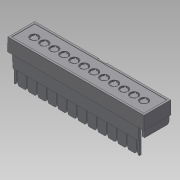
# Autodesk Inventor part: D2MG guard
Saved by Autodesk Inventor 2018.2 (Build 222227000, 227)
## iProperties
Created: 2015-02-09
Part Number: D2MG guard
Material: Типовые
Document SubType Name: Modeling
Designer: Abbath
Density: 1 g/cm^3
Appearance: По умолчанию
Mass: 2.0666 g
Surface Area: 34.2818 cm^2
Volume: 2.0666 cm^3
Author: Abbath
Autodesk Inventor part; units mm, degrees
ref_plane "YZ Plane" through (0, 0, 0) normal (1, 0, 0) x (0, 1, 0)
ref_plane "XZ Plane" through (0, 0, 0) normal (0, 1, 0) x (-1, 0, 0)
sketch "Эскиз1" plane through (0, 0, 0) normal (0, 0, 1) x (1, 0, 0)
  line L0 (-34.8, 6.95) -> (34.8, 6.95)
  line L1 (34.8, 6.95) -> (34.8, -6.95)
  line L2 (34.8, -6.95) -> (-34.8, -6.95)
  line L3 (-34.8, -6.95) -> (-34.8, 6.95)
  point P0 (0, 0)
  point P1 (34.8, 0)
  point P2 (0, 6.95)
  dimension "d0" = 13.9
  dimension "d1" = 69.6
  constraints: 8 end point, 2 midpoint, 2 parallel, 1 horizontal, 1 horizontal alignment, 1 perpendicular, 1 vertical alignment
  measures "d0" distance between parallel lines of L2 L0
  measures "d1" distance between parallel lines of L1 L3
ref_plane "РабПлоскость1" through (0, 0, 6.5) normal (0, 0, 1) x (1, 0, 0)
sketch "Эскиз2" plane through (0, 0, 6.5) normal (0, 0, 1) x (1, 0, 0)
  line L0 (-34.685, 6.85) -> (34.685, 6.85)
  line L1 (34.685, 6.85) -> (34.685, -6.95)
  line L2 (34.685, -6.95) -> (-34.685, -6.95)
  line L3 (-34.685, -6.95) -> (-34.685, 6.85)
  line L4 (34.8, -6.95) -> (-34.8, -6.95) projected
  point P0 (0, 0)
  point P1 (0, 6.85)
  point P2 (0, -6.95)
  dimension "d3" = 13.8
  dimension "d4" = 69.37
  constraints: 8 end point, 2 midpoint, 2 parallel, 1 collinear, 1 horizontal, 1 perpendicular, 1 vertical alignment
  measures "d3" distance between parallel lines of L2 L0
  measures "d4" distance between parallel lines of L1 L3
loft "Лофт1" add profiles "Эскиз1", "Эскиз2"
sketch "Эскиз3" plane through (-34.8, -6.95, 0) normal (0, -1, 0) x (1, 0, 0)
  line L0 (32.55, 7.5) -> (37.05, 7.5)
  line L1 (37.05, 7.5) -> (37.05, 1)
  line L2 (37.05, 1) -> (32.55, 1)
  line L3 (32.55, 1) -> (32.55, 7.5)
  line L4 (69.6, 0) -> (0, 0) projected
  line L5 (69.485, 6.5) -> (0.115, 6.5) construction
  point P0 (34.8, 0)
  point P1 (34.8, 1)
  point P2 (34.8, 0)
  dimension "d9" = 1
  dimension "d10" = 5.5
  dimension "d11" = 4.5
  constraints: 8 end point, 2 midpoint, 2 parallel, 1 horizontal, 1 perpendicular, 1 vertical alignment
  measures "d9" distance between parallel lines of L5 L0
  measures "d10" distance between parallel lines of L2 L5
  measures "d11" distance between parallel lines of L1 L3
extrude "Выдавливание1" cut sketch "Эскиз3" against normal blind 0.5
sketch "Эскиз4" plane through (-34.685, 6.85, 6.5) normal (0, 0, 1) x (1, 0, 0)
  line L0 (32.435, -13.8) -> (32.435, -13.3) construction
  line L1 (32.435, -13.3) -> (36.935, -13.3) construction
  line L2 (36.935, -13.3) -> (36.935, -13.8) construction
  line L3 (69.37, -13.8) -> (36.935, -13.8) construction
  line L4 (69.37, 0) -> (69.37, -13.8) construction
  line L5 (0, 0) -> (69.37, 0) construction
  line L6 (0, -13.8) -> (0, 0) construction
  line L7 (32.435, -13.8) -> (0, -13.8) construction
  line L8 (32.435, -13.8) -> (32.435, -13.3) construction
  line L9 (32.435, -13.3) -> (36.935, -13.3) construction
  line L10 (36.935, -13.3) -> (36.935, -13.8) construction
  line L11 (69.37, -13.8) -> (36.935, -13.8) construction
  line L12 (69.37, 0) -> (69.37, -13.8) construction
  line L13 (0, 0) -> (69.37, 0) construction
  line L14 (0, -13.8) -> (0, 0) construction
  line L15 (32.435, -13.8) -> (0, -13.8) construction
  line L16 (1, -1) -> (68.37, -1)
  line L17 (68.37, -1) -> (68.37, -12.8)
  line L18 (68.37, -12.8) -> (1, -12.8)
  line L19 (1, -12.8) -> (1, -1)
  dimension "d103" = 1
  dimension "d104" = 1
  dimension "d105" = 1
  dimension "d106" = 1
  constraints: 8 end point, 2 parallel, 1 horizontal, 1 perpendicular
  measures "d103" distance between parallel lines of L6 L19
  measures "d104" distance between parallel lines of L4 L17
  measures "d105" distance between parallel lines of L5 L16
  measures "d106" distance between parallel lines of L3 L18
extrude "Выдавливание2" cut sketch "Эскиз4" against normal blind 0.2
sketch "Эскиз5" plane through (-34.685, 6.85, 6.3) normal (0, 0, 1) x (1, 0, 0)
  line L0 (-0.115, 0.1) -> (69.485, 0.1) construction
  line L1 (34.685, 0.1) -> (34.685, -13.8) construction
  line L2 (69.485, -13.8) -> (-0.115, -13.8) construction
  line L3 (34.685, -6.85) -> (81.7504, -6.85) construction
  circle A0 centre (37.225, -6.85) radius 2.1
  circle A1 centre (42.305, -6.85) radius 2.1
  circle A2 centre (47.385, -6.85) radius 2.1
  circle A3 centre (52.465, -6.85) radius 2.1
  circle A4 centre (57.545, -6.85) radius 2.1
  circle A5 centre (62.625, -6.85) radius 2.1
  circle A6 centre (32.145, -6.85) radius 2.1
  circle A7 centre (37.225, -6.85) radius 2.1
  circle A8 centre (42.305, -6.85) radius 2.1
  circle A9 centre (47.385, -6.85) radius 2.1
  circle A10 centre (52.465, -6.85) radius 2.1
  circle A11 centre (57.545, -6.85) radius 2.1
  circle A12 centre (27.065, -6.85) radius 2.1
  circle A13 centre (32.145, -6.85) radius 2.1
  circle A14 centre (37.225, -6.85) radius 2.1
  circle A15 centre (42.305, -6.85) radius 2.1
  circle A16 centre (47.385, -6.85) radius 2.1
  circle A17 centre (52.465, -6.85) radius 2.1
  circle A18 centre (21.985, -6.85) radius 2.1
  circle A19 centre (27.065, -6.85) radius 2.1
  circle A20 centre (32.145, -6.85) radius 2.1
  circle A21 centre (37.225, -6.85) radius 2.1
  circle A22 centre (42.305, -6.85) radius 2.1
  circle A23 centre (47.385, -6.85) radius 2.1
  circle A24 centre (16.905, -6.85) radius 2.1
  circle A25 centre (21.985, -6.85) radius 2.1
  circle A26 centre (27.065, -6.85) radius 2.1
  circle A27 centre (32.145, -6.85) radius 2.1
  circle A28 centre (37.225, -6.85) radius 2.1
  circle A29 centre (42.305, -6.85) radius 2.1
  circle A30 centre (11.825, -6.85) radius 2.1
  circle A31 centre (16.905, -6.85) radius 2.1
  circle A32 centre (21.985, -6.85) radius 2.1
  circle A33 centre (27.065, -6.85) radius 2.1
  circle A34 centre (32.145, -6.85) radius 2.1
  circle A35 centre (37.225, -6.85) radius 2.1
  circle A36 centre (6.745, -6.85) radius 2.1
  circle A37 centre (11.825, -6.85) radius 2.1
  circle A38 centre (16.905, -6.85) radius 2.1
  circle A39 centre (21.985, -6.85) radius 2.1
  circle A40 centre (27.065, -6.85) radius 2.1
  circle A41 centre (32.145, -6.85) radius 2.1
  line L4 (32.145, -6.85) -> (37.225, -6.85) construction
  dimension "d107" = 4.2
  dimension "d110" = 5.08
  dimension "d113" = 5.08
  constraints: 42 centre point, 6 end point, 5 midpoint, 3 horizontal, 1 collinear, 1 point on line, 82 other
  measures "d107" diameter of A0
  measures "d110" distance of A0.centre A1.centre
  measures "d113" distance of A0.centre A6.centre
extrude "Выдавливание3" cut sketch "Эскиз5" against normal blind 0.3
sketch "Эскиз6" plane through (-12.7, 0, 6) normal (0, 0, 1) x (1, 0, 0)
  circle A0 centre (-15.24, 0) radius 2.1 construction
  circle A1 centre (-15.24, 0) radius 2.1 projected
  line L0 (-17.3106, 0.35) -> (-16.6986, 0.35)
  line L1 (-17.3106, -0.35) -> (-16.6986, -0.35)
  line L2 (-15.24, 0) -> (-17.34, 0) construction
  line L3 (-17.0605, 0.35) -> (-17.0605, -0.35) construction
  line L4 (-14.5078, -1.9682) -> (-14.8138, -1.4382)
  line L5 (-13.9016, -1.6182) -> (-14.2076, -1.0882)
  line L6 (-13.9016, 1.6182) -> (-14.2076, 1.0882)
  line L7 (-14.5078, 1.9682) -> (-14.8138, 1.4382)
  arc A2 (-14.8138, 1.4382) -> (-16.6986, 0.35) centre (-15.24, 0) ccw
  arc A3 (-14.5078, 1.9682) -> (-17.3106, 0.35) centre (-15.24, 0) ccw
  arc A4 (-17.3106, -0.35) -> (-14.5078, -1.9682) centre (-15.24, 0) ccw
  arc A5 (-13.9016, -1.6182) -> (-13.9016, 1.6182) centre (-15.24, 0) ccw
  arc A6 (-16.6986, -0.35) -> (-14.8138, -1.4382) centre (-15.24, 0) ccw
  arc A7 (-14.2076, -1.0882) -> (-14.2076, 1.0882) centre (-15.24, 0) ccw
  line L8 (-9.4278, 1.9682) -> (-9.7338, 1.4382)
  line L9 (-9.4278, -1.9682) -> (-9.7338, -1.4382)
  arc A8 (-9.7338, 1.4382) -> (-11.6186, 0.35) centre (-10.16, 0) ccw
  arc A9 (-9.4278, 1.9682) -> (-12.2306, 0.35) centre (-10.16, 0) ccw
  arc A10 (-11.6186, -0.35) -> (-9.7338, -1.4382) centre (-10.16, 0) ccw
  arc A11 (-12.2306, -0.35) -> (-9.4278, -1.9682) centre (-10.16, 0) ccw
  line L10 (-10.16, 0) -> (-12.26, 0) construction
  line L11 (-11.9805, 0.35) -> (-11.9805, -0.35) construction
  line L12 (-12.2306, -0.35) -> (-11.6186, -0.35)
  line L13 (-12.2306, 0.35) -> (-11.6186, 0.35)
  line L14 (-8.8216, -1.6182) -> (-9.1276, -1.0882)
  arc A12 (-9.1276, -1.0882) -> (-9.1276, 1.0882) centre (-10.16, 0) ccw
  arc A13 (-8.8216, -1.6182) -> (-8.8216, 1.6182) centre (-10.16, 0) ccw
  line L15 (-8.8216, 1.6182) -> (-9.1276, 1.0882)
  line L16 (-4.3478, 1.9682) -> (-4.6538, 1.4382)
  line L17 (-4.3478, -1.9682) -> (-4.6538, -1.4382)
  arc A14 (-4.6538, 1.4382) -> (-6.5386, 0.35) centre (-5.08, 0) ccw
  arc A15 (-4.3478, 1.9682) -> (-7.1506, 0.35) centre (-5.08, 0) ccw
  arc A16 (-6.5386, -0.35) -> (-4.6538, -1.4382) centre (-5.08, 0) ccw
  arc A17 (-7.1506, -0.35) -> (-4.3478, -1.9682) centre (-5.08, 0) ccw
  line L18 (-5.08, 0) -> (-7.18, 0) construction
  line L19 (-6.9005, 0.35) -> (-6.9005, -0.35) construction
  line L20 (-7.1506, -0.35) -> (-6.5386, -0.35)
  line L21 (-7.1506, 0.35) -> (-6.5386, 0.35)
  line L22 (-3.7416, -1.6182) -> (-4.0476, -1.0882)
  arc A18 (-4.0476, -1.0882) -> (-4.0476, 1.0882) centre (-5.08, 0) ccw
  arc A19 (-3.7416, -1.6182) -> (-3.7416, 1.6182) centre (-5.08, 0) ccw
  line L23 (-3.7416, 1.6182) -> (-4.0476, 1.0882)
  line L24 (0.7322, 1.9682) -> (0.4262, 1.4382)
  line L25 (0.7322, -1.9682) -> (0.4262, -1.4382)
  arc A20 (0.4262, 1.4382) -> (-1.4586, 0.35) centre (0, 0) ccw
  arc A21 (0.7322, 1.9682) -> (-2.0706, 0.35) centre (0, 0) ccw
  arc A22 (-1.4586, -0.35) -> (0.4262, -1.4382) centre (0, 0) ccw
  arc A23 (-2.0706, -0.35) -> (0.7322, -1.9682) centre (0, 0) ccw
  line L26 (0, 0) -> (-2.1, 0) construction
  line L27 (-1.8205, 0.35) -> (-1.8205, -0.35) construction
  line L28 (-2.0706, -0.35) -> (-1.4586, -0.35)
  line L29 (-2.0706, 0.35) -> (-1.4586, 0.35)
  line L30 (1.3384, -1.6182) -> (1.0324, -1.0882)
  arc A24 (1.0324, -1.0882) -> (1.0324, 1.0882) centre (0, 0) ccw
  arc A25 (1.3384, -1.6182) -> (1.3384, 1.6182) centre (0, 0) ccw
  line L31 (1.3384, 1.6182) -> (1.0324, 1.0882)
  line L32 (5.8122, 1.9682) -> (5.5062, 1.4382)
  line L33 (5.8122, -1.9682) -> (5.5062, -1.4382)
  arc A26 (5.5062, 1.4382) -> (3.6214, 0.35) centre (5.08, 0) ccw
  arc A27 (5.8122, 1.9682) -> (3.0094, 0.35) centre (5.08, 0) ccw
  arc A28 (3.6214, -0.35) -> (5.5062, -1.4382) centre (5.08, 0) ccw
  arc A29 (3.0094, -0.35) -> (5.8122, -1.9682) centre (5.08, 0) ccw
  line L34 (5.08, 0) -> (2.98, 0) construction
  line L35 (3.2595, 0.35) -> (3.2595, -0.35) construction
  line L36 (3.0094, -0.35) -> (3.6214, -0.35)
  line L37 (3.0094, 0.35) -> (3.6214, 0.35)
  line L38 (6.4184, -1.6182) -> (6.1124, -1.0882)
  arc A30 (6.1124, -1.0882) -> (6.1124, 1.0882) centre (5.08, 0) ccw
  arc A31 (6.4184, -1.6182) -> (6.4184, 1.6182) centre (5.08, 0) ccw
  line L39 (6.4184, 1.6182) -> (6.1124, 1.0882)
  line L40 (10.8922, 1.9682) -> (10.5862, 1.4382)
  line L41 (10.8922, -1.9682) -> (10.5862, -1.4382)
  arc A32 (10.5862, 1.4382) -> (8.7014, 0.35) centre (10.16, 0) ccw
  arc A33 (10.8922, 1.9682) -> (8.0894, 0.35) centre (10.16, 0) ccw
  arc A34 (8.7014, -0.35) -> (10.5862, -1.4382) centre (10.16, 0) ccw
  arc A35 (8.0894, -0.35) -> (10.8922, -1.9682) centre (10.16, 0) ccw
  line L42 (10.16, 0) -> (8.06, 0) construction
  line L43 (8.3395, 0.35) -> (8.3395, -0.35) construction
  line L44 (8.0894, -0.35) -> (8.7014, -0.35)
  line L45 (8.0894, 0.35) -> (8.7014, 0.35)
  line L46 (11.4984, -1.6182) -> (11.1924, -1.0882)
  arc A36 (11.1924, -1.0882) -> (11.1924, 1.0882) centre (10.16, 0) ccw
  arc A37 (11.4984, -1.6182) -> (11.4984, 1.6182) centre (10.16, 0) ccw
  line L47 (11.4984, 1.6182) -> (11.1924, 1.0882)
  line L48 (15.9722, 1.9682) -> (15.6662, 1.4382)
  line L49 (15.9722, -1.9682) -> (15.6662, -1.4382)
  arc A38 (15.6662, 1.4382) -> (13.7814, 0.35) centre (15.24, 0) ccw
  arc A39 (15.9722, 1.9682) -> (13.1694, 0.35) centre (15.24, 0) ccw
  arc A40 (13.7814, -0.35) -> (15.6662, -1.4382) centre (15.24, 0) ccw
  arc A41 (13.1694, -0.35) -> (15.9722, -1.9682) centre (15.24, 0) ccw
  line L50 (15.24, 0) -> (13.14, 0) construction
  line L51 (13.4195, 0.35) -> (13.4195, -0.35) construction
  line L52 (13.1694, -0.35) -> (13.7814, -0.35)
  line L53 (13.1694, 0.35) -> (13.7814, 0.35)
  line L54 (16.5784, -1.6182) -> (16.2724, -1.0882)
  arc A42 (16.2724, -1.0882) -> (16.2724, 1.0882) centre (15.24, 0) ccw
  arc A43 (16.5784, -1.6182) -> (16.5784, 1.6182) centre (15.24, 0) ccw
  line L55 (16.5784, 1.6182) -> (16.2724, 1.0882)
  line L56 (21.0522, 1.9682) -> (20.7462, 1.4382)
  line L57 (21.0522, -1.9682) -> (20.7462, -1.4382)
  arc A44 (20.7462, 1.4382) -> (18.8614, 0.35) centre (20.32, 0) ccw
  arc A45 (21.0522, 1.9682) -> (18.2494, 0.35) centre (20.32, 0) ccw
  arc A46 (18.8614, -0.35) -> (20.7462, -1.4382) centre (20.32, 0) ccw
  arc A47 (18.2494, -0.35) -> (21.0522, -1.9682) centre (20.32, 0) ccw
  line L58 (20.32, 0) -> (18.22, 0) construction
  line L59 (18.4995, 0.35) -> (18.4995, -0.35) construction
  line L60 (18.2494, -0.35) -> (18.8614, -0.35)
  line L61 (18.2494, 0.35) -> (18.8614, 0.35)
  line L62 (21.6584, -1.6182) -> (21.3524, -1.0882)
  arc A48 (21.3524, -1.0882) -> (21.3524, 1.0882) centre (20.32, 0) ccw
  arc A49 (21.6584, -1.6182) -> (21.6584, 1.6182) centre (20.32, 0) ccw
  line L63 (21.6584, 1.6182) -> (21.3524, 1.0882)
  line L64 (26.1322, 1.9682) -> (25.8262, 1.4382)
  line L65 (26.1322, -1.9682) -> (25.8262, -1.4382)
  arc A50 (25.8262, 1.4382) -> (23.9414, 0.35) centre (25.4, 0) ccw
  arc A51 (26.1322, 1.9682) -> (23.3294, 0.35) centre (25.4, 0) ccw
  arc A52 (23.9414, -0.35) -> (25.8262, -1.4382) centre (25.4, 0) ccw
  arc A53 (23.3294, -0.35) -> (26.1322, -1.9682) centre (25.4, 0) ccw
  line L66 (25.4, 0) -> (23.3, 0) construction
  line L67 (23.5795, 0.35) -> (23.5795, -0.35) construction
  line L68 (23.3294, -0.35) -> (23.9414, -0.35)
  line L69 (23.3294, 0.35) -> (23.9414, 0.35)
  line L70 (26.7384, -1.6182) -> (26.4324, -1.0882)
  arc A54 (26.4324, -1.0882) -> (26.4324, 1.0882) centre (25.4, 0) ccw
  arc A55 (26.7384, -1.6182) -> (26.7384, 1.6182) centre (25.4, 0) ccw
  line L71 (26.7384, 1.6182) -> (26.4324, 1.0882)
  line L72 (31.2122, 1.9682) -> (30.9062, 1.4382)
  line L73 (31.2122, -1.9682) -> (30.9062, -1.4382)
  arc A56 (30.9062, 1.4382) -> (29.0214, 0.35) centre (30.48, 0) ccw
  arc A57 (31.2122, 1.9682) -> (28.4094, 0.35) centre (30.48, 0) ccw
  arc A58 (29.0214, -0.35) -> (30.9062, -1.4382) centre (30.48, 0) ccw
  arc A59 (28.4094, -0.35) -> (31.2122, -1.9682) centre (30.48, 0) ccw
  line L74 (30.48, 0) -> (28.38, 0) construction
  line L75 (28.6595, 0.35) -> (28.6595, -0.35) construction
  line L76 (28.4094, -0.35) -> (29.0214, -0.35)
  line L77 (28.4094, 0.35) -> (29.0214, 0.35)
  line L78 (31.8184, -1.6182) -> (31.5124, -1.0882)
  arc A60 (31.5124, -1.0882) -> (31.5124, 1.0882) centre (30.48, 0) ccw
  arc A61 (31.8184, -1.6182) -> (31.8184, 1.6182) centre (30.48, 0) ccw
  line L79 (31.8184, 1.6182) -> (31.5124, 1.0882)
  line L80 (36.2922, 1.9682) -> (35.9862, 1.4382)
  line L81 (36.2922, -1.9682) -> (35.9862, -1.4382)
  arc A62 (35.9862, 1.4382) -> (34.1014, 0.35) centre (35.56, 0) ccw
  arc A63 (36.2922, 1.9682) -> (33.4894, 0.35) centre (35.56, 0) ccw
  arc A64 (34.1014, -0.35) -> (35.9862, -1.4382) centre (35.56, 0) ccw
  arc A65 (33.4894, -0.35) -> (36.2922, -1.9682) centre (35.56, 0) ccw
  line L82 (35.56, 0) -> (33.46, 0) construction
  line L83 (33.7395, 0.35) -> (33.7395, -0.35) construction
  line L84 (33.4894, -0.35) -> (34.1014, -0.35)
  line L85 (33.4894, 0.35) -> (34.1014, 0.35)
  line L86 (36.8984, -1.6182) -> (36.5924, -1.0882)
  arc A66 (36.5924, -1.0882) -> (36.5924, 1.0882) centre (35.56, 0) ccw
  arc A67 (36.8984, -1.6182) -> (36.8984, 1.6182) centre (35.56, 0) ccw
  line L87 (36.8984, 1.6182) -> (36.5924, 1.0882)
  line L88 (41.3722, 1.9682) -> (41.0662, 1.4382)
  line L89 (41.3722, -1.9682) -> (41.0662, -1.4382)
  arc A68 (41.0662, 1.4382) -> (39.1814, 0.35) centre (40.64, 0) ccw
  arc A69 (41.3722, 1.9682) -> (38.5694, 0.35) centre (40.64, 0) ccw
  arc A70 (39.1814, -0.35) -> (41.0662, -1.4382) centre (40.64, 0) ccw
  arc A71 (38.5694, -0.35) -> (41.3722, -1.9682) centre (40.64, 0) ccw
  line L90 (40.64, 0) -> (38.54, 0) construction
  line L91 (38.8195, 0.35) -> (38.8195, -0.35) construction
  line L92 (38.5694, -0.35) -> (39.1814, -0.35)
  line L93 (38.5694, 0.35) -> (39.1814, 0.35)
  line L94 (41.9784, -1.6182) -> (41.6724, -1.0882)
  arc A72 (41.6724, -1.0882) -> (41.6724, 1.0882) centre (40.64, 0) ccw
  arc A73 (41.9784, -1.6182) -> (41.9784, 1.6182) centre (40.64, 0) ccw
  line L95 (41.9784, 1.6182) -> (41.6724, 1.0882)
  point P0 (-17.0605, 0)
  point P1 (-14.6329, -1.7516)
  point P2 (-14.0266, -1.4016)
  point P3 (-14.0266, 1.4016)
  point P4 (-14.6329, 1.7516)
  point P5 (-9.5529, -1.7516)
  point P6 (-9.5529, 1.7516)
  point P7 (-11.9805, 0)
  point P8 (-8.9466, 1.4016)
  point P9 (-8.9466, -1.4016)
  point P10 (-4.4729, -1.7516)
  point P11 (-4.4729, 1.7516)
  point P12 (-6.9005, 0)
  point P13 (-3.8666, 1.4016)
  point P14 (-3.8666, -1.4016)
  point P15 (0.6071, -1.7516)
  point P16 (0.6071, 1.7516)
  point P17 (-1.8205, 0)
  point P18 (1.2134, 1.4016)
  point P19 (1.2134, -1.4016)
  point P20 (5.6871, -1.7516)
  point P21 (5.6871, 1.7516)
  point P22 (3.2595, 0)
  point P23 (6.2934, 1.4016)
  point P24 (6.2934, -1.4016)
  point P25 (10.7671, -1.7516)
  point P26 (10.7671, 1.7516)
  point P27 (8.3395, 0)
  point P28 (11.3734, 1.4016)
  point P29 (11.3734, -1.4016)
  point P30 (15.8471, -1.7516)
  point P31 (15.8471, 1.7516)
  point P32 (13.4195, 0)
  point P33 (16.4534, 1.4016)
  point P34 (16.4534, -1.4016)
  point P35 (20.9271, -1.7516)
  point P36 (20.9271, 1.7516)
  point P37 (18.4995, 0)
  point P38 (21.5334, 1.4016)
  point P39 (21.5334, -1.4016)
  point P40 (26.0071, -1.7516)
  point P41 (26.0071, 1.7516)
  point P42 (23.5795, 0)
  point P43 (26.6134, 1.4016)
  point P44 (26.6134, -1.4016)
  point P45 (31.0871, -1.7516)
  point P46 (31.0871, 1.7516)
  point P47 (28.6595, 0)
  point P48 (31.6934, 1.4016)
  point P49 (31.6934, -1.4016)
  point P50 (36.1671, -1.7516)
  point P51 (36.1671, 1.7516)
  point P52 (33.7395, 0)
  point P53 (36.7734, 1.4016)
  point P54 (36.7734, -1.4016)
  point P55 (41.2471, -1.7516)
  point P56 (41.2471, 1.7516)
  point P57 (38.8195, 0)
  point P58 (41.8534, 1.4016)
  point P59 (41.8534, -1.4016)
  dimension "d117" = 0.7
  dimension "d120" = 360
  dimension "d131" = 5.08
  constraints: 192 end point, 147 point on circle, 84 point on line, 72 centre point, 13 coincident, 3 horizontal, 1 collinear, 1 midpoint, 1 parallel, 1 perpendicular, 431 other
  measures "d117" distance between parallel lines of L1 L0
  measures "d131" distance of A3.centre A9.centre
extrude "Выдавливание4" cut sketch "Эскиз6" against normal through all contours A1 L5 A7 L6 | L7 A2 L0 A1 | A1 L1 A6 L4 | L8 A8 L13 A9 | A11 L12 A10 L9 | L14 A12 L15 A13 | L16 A14 L21 A15 | A17 L20 A16 L17 | L22 A18 L23 A19 | L24 A20 L29 A21 | A23 L28 A22 L25 | L30 A24 L31 A25 | L32 A26 L37 A27 | A29 L36 A28 L33 | L38 A30 L39 A31 | L40 A32 L45 A33 | A35 L44 A34 L41 | L46 A36 L47 A37 | L48 A38 L53 A39 | A41 L52 A40 L49 | L54 A42 L55 A43 | L56 A44 L61 A45 | A47 L60 A46 L57 | L62 A48 L63 A49 | L64 A50 L69 A51 | A53 L68 A52 L65 | L70 A54 L71 A55 | L72 A56 L77 A57 | A59 L76 A58 L73 | L78 A60 L79 A61 | L80 A62 L85 A63 | A65 L84 A64 L81 | L86 A66 L87 A67 | L88 A68 L93 A69 | A71 L92 A70 L89 | L94 A72 L95 A73
sketch "Эскиз7" plane through (34.8, 6.95, 0) normal (0, 0, -1) x (-1, 0, 0)
  line L0 (2.9, 0) -> (66.7, 0)
  line L1 (66.7, 0) -> (66.7, -1.5)
  line L2 (66.7, -1.5) -> (2.9, -1.5)
  line L3 (2.9, -1.5) -> (2.9, 0)
  line L4 (69.6, 0) -> (0, 0) construction
  point P0 (34.8, -6.95)
  point P1 (34.8, -1.5)
  dimension "d39" = 1.5
  dimension "d40" = 63.8
  constraints: 8 end point, 2 parallel, 1 collinear, 1 horizontal, 1 midpoint, 1 perpendicular, 1 vertical alignment
  measures "d39" distance between parallel lines of L2 L4
  measures "d40" distance between parallel lines of L1 L3
extrude "Выдавливание5" add sketch "Эскиз7" along normal blind 12.9
sketch "Эскиз8" plane through (0, 0, 0) normal (1, 0, 0) x (0, 1, 0)
  line L0 (6.33, -12.9) -> (6.42, -5.85)
  line L1 (6.42, -5.85) -> (6.95, -5.85)
  line L2 (5.45, 0) -> (5.45, -12.9) projected
  line L3 (6.95, -5.85) -> (6.95, -12.9)
  line L4 (6.95, -12.9) -> (6.33, -12.9)
  line L5 (6.95, -12.9) -> (5.45, -12.9) construction
  line L6 (6.95, 0) -> (6.95, -12.9) construction
  point P0 (0, 0)
  dimension "d43" = 0.53
  dimension "d44" = 0.88
  dimension "d45" = 7.05
  constraints: 8 end point, 3 perpendicular, 2 collinear
  measures "d43" distance from line of L0.end L3
  measures "d44" distance from line of L0.start L2
  measures "d45" distance from line of L1 L0.start
extrude "Выдавливание6" cut sketch "Эскиз8" along normal through all both and the other way through all
sketch "Эскиз10" plane through (34.8, -6.95, 0) normal (0, 0, -1) x (-1, 0, 0)
  line L0 (67.3, 12.4) -> (2.3, 12.4)
  line L1 (2.3, 12.4) -> (2.3, 1.5)
  line L2 (2.3, 1.5) -> (67.3, 1.5)
  line L3 (67.3, 1.5) -> (67.3, 12.4)
  line L4 (69.6, 0) -> (69.6, 13.9) projected
  line L5 (0, 0) -> (69.6, 0) projected
  line L6 (0, 13.9) -> (0, 0) projected
  line L7 (2.9, 12.4) -> (66.7, 12.4) projected
  point P0 (34.8, 6.95)
  point P1 (45.71, 12.4)
  point P2 (34.8, 1.5)
  dimension "d63" = 1.5
  dimension "d70" = 65
  constraints: 8 end point, 2 parallel, 1 collinear, 1 horizontal, 1 midpoint, 1 perpendicular, 1 vertical alignment
  measures "d63" distance between parallel lines of L5 L2
  measures "d70" distance between parallel lines of L1 L3
extrude "Выдавливание8" cut sketch "Эскиз10" against normal blind 5
sketch "Эскиз17" plane through (-31.9, 6.42, -5.85) normal (0, 0.9999185, -0.0127649) x (1, 0, 0)
  line L0 (0.52, 7.0618) -> (1.17, 5.5381)
  line L1 (1.17, 5.5381) -> (1.17, -0.0455)
  line L2 (1.17, -0.0455) -> (1.67, -0.0455)
  line L3 (1.67, -0.0455) -> (1.67, 5.5381)
  line L4 (1.67, 5.5381) -> (2.32, 7.0618)
  line L5 (0.52, 7.0618) -> (2.32, 7.0618)
  line L6 (1.42, 0) -> (1.42, 8.247) construction
  line L7 (1.17, 0.6294) -> (1.67, 0.6294) construction
  line L8 (0, -5.8371) -> (0, 7.0618) construction
  line L9 (0, 4.1598) -> (63.8, 4.1598) construction
  line L10 (63.8, -5.8371) -> (63.8, 7.0618) construction
  line L11 (31.65, 5.5381) -> (32.15, 5.5381) construction
  line L12 (0.52, 7.0618) -> (2.32, 7.0618) construction
  line L13 (5.6, 7.0618) -> (7.4, 7.0618) construction
  line L14 (10.68, 7.0618) -> (12.48, 7.0618) construction
  line L15 (0.52, 7.0618) -> (2.32, 7.0618) construction
  line L16 (1.17, -0.0455) -> (1.67, -0.0455) construction
  line L17 (63.8, 0) -> (0, 0) projected
  line L18 (1.17, 0) -> (1.67, 0)
  line L19 (6.75, 5.5381) -> (7.4, 7.0618)
  line L20 (5.6, 7.0618) -> (6.25, 5.5381)
  line L21 (5.6, 7.0618) -> (7.4, 7.0618)
  line L22 (5.6, 7.0618) -> (7.4, 7.0618) construction
  line L23 (6.25, 0.6294) -> (6.75, 0.6294) construction
  line L24 (6.75, -0.0455) -> (6.75, 5.5381)
  line L25 (6.25, 5.5381) -> (6.25, -0.0455)
  line L26 (6.25, 0) -> (6.75, 0)
  line L27 (6.25, -0.0455) -> (6.75, -0.0455)
  line L28 (6.25, -0.0455) -> (6.75, -0.0455) construction
  line L29 (36.73, 5.5381) -> (37.23, 5.5381) construction
  line L30 (11.83, 5.5381) -> (12.48, 7.0618)
  line L31 (10.68, 7.0618) -> (11.33, 5.5381)
  line L32 (10.68, 7.0618) -> (12.48, 7.0618)
  line L33 (10.68, 7.0618) -> (12.48, 7.0618) construction
  line L34 (11.33, 0.6294) -> (11.83, 0.6294) construction
  line L35 (11.83, -0.0455) -> (11.83, 5.5381)
  line L36 (11.33, 5.5381) -> (11.33, -0.0455)
  line L37 (11.33, 0) -> (11.83, 0)
  line L38 (11.33, -0.0455) -> (11.83, -0.0455)
  line L39 (11.33, -0.0455) -> (11.83, -0.0455) construction
  line L40 (41.81, 5.5381) -> (42.31, 5.5381) construction
  line L41 (16.91, 5.5381) -> (17.56, 7.0618)
  line L42 (15.76, 7.0618) -> (16.41, 5.5381)
  line L43 (15.76, 7.0618) -> (17.56, 7.0618)
  line L44 (15.76, 7.0618) -> (17.56, 7.0618) construction
  line L45 (16.41, 0.6294) -> (16.91, 0.6294) construction
  line L46 (16.91, -0.0455) -> (16.91, 5.5381)
  line L47 (16.41, 5.5381) -> (16.41, -0.0455)
  line L48 (16.41, 0) -> (16.91, 0)
  line L49 (16.41, -0.0455) -> (16.91, -0.0455)
  line L50 (16.41, -0.0455) -> (16.91, -0.0455) construction
  line L51 (46.89, 5.5381) -> (47.39, 5.5381) construction
  line L52 (21.99, 5.5381) -> (22.64, 7.0618)
  line L53 (20.84, 7.0618) -> (21.49, 5.5381)
  line L54 (20.84, 7.0618) -> (22.64, 7.0618)
  line L55 (20.84, 7.0618) -> (22.64, 7.0618) construction
  line L56 (21.49, 0.6294) -> (21.99, 0.6294) construction
  line L57 (21.99, -0.0455) -> (21.99, 5.5381)
  line L58 (21.49, 5.5381) -> (21.49, -0.0455)
  line L59 (21.49, 0) -> (21.99, 0)
  line L60 (21.49, -0.0455) -> (21.99, -0.0455)
  line L61 (21.49, -0.0455) -> (21.99, -0.0455) construction
  line L62 (51.97, 5.5381) -> (52.47, 5.5381) construction
  line L63 (27.07, 5.5381) -> (27.72, 7.0618)
  line L64 (25.92, 7.0618) -> (26.57, 5.5381)
  line L65 (25.92, 7.0618) -> (27.72, 7.0618)
  line L66 (25.92, 7.0618) -> (27.72, 7.0618) construction
  line L67 (26.57, 0.6294) -> (27.07, 0.6294) construction
  line L68 (27.07, -0.0455) -> (27.07, 5.5381)
  line L69 (26.57, 5.5381) -> (26.57, -0.0455)
  line L70 (26.57, 0) -> (27.07, 0)
  line L71 (26.57, -0.0455) -> (27.07, -0.0455)
  line L72 (26.57, -0.0455) -> (27.07, -0.0455) construction
  line L73 (57.05, 5.5381) -> (57.55, 5.5381) construction
  line L74 (32.15, 5.5381) -> (32.8, 7.0618)
  line L75 (31, 7.0618) -> (31.65, 5.5381)
  line L76 (31, 7.0618) -> (32.8, 7.0618)
  line L77 (31, 7.0618) -> (32.8, 7.0618) construction
  line L78 (31.65, 0.6294) -> (32.15, 0.6294) construction
  line L79 (32.15, -0.0455) -> (32.15, 5.5381)
  line L80 (31.65, 5.5381) -> (31.65, -0.0455)
  line L81 (31.65, 0) -> (32.15, 0)
  line L82 (31.65, -0.0455) -> (32.15, -0.0455)
  line L83 (31.65, -0.0455) -> (32.15, -0.0455) construction
  line L84 (62.13, 5.5381) -> (62.63, 5.5381) construction
  line L85 (37.23, 5.5381) -> (37.88, 7.0618)
  line L86 (36.08, 7.0618) -> (36.73, 5.5381)
  line L87 (36.08, 7.0618) -> (37.88, 7.0618)
  line L88 (36.08, 7.0618) -> (37.88, 7.0618) construction
  line L89 (36.73, 0.6294) -> (37.23, 0.6294) construction
  line L90 (37.23, -0.0455) -> (37.23, 5.5381)
  line L91 (36.73, 5.5381) -> (36.73, -0.0455)
  line L92 (36.73, 0) -> (37.23, 0)
  line L93 (36.73, -0.0455) -> (37.23, -0.0455)
  line L94 (36.73, -0.0455) -> (37.23, -0.0455) construction
  line L95 (67.21, 5.5381) -> (67.71, 5.5381) construction
  line L96 (42.31, 5.5381) -> (42.96, 7.0618)
  line L97 (41.16, 7.0618) -> (41.81, 5.5381)
  line L98 (41.16, 7.0618) -> (42.96, 7.0618)
  line L99 (41.16, 7.0618) -> (42.96, 7.0618) construction
  line L100 (41.81, 0.6294) -> (42.31, 0.6294) construction
  line L101 (42.31, -0.0455) -> (42.31, 5.5381)
  line L102 (41.81, 5.5381) -> (41.81, -0.0455)
  line L103 (41.81, 0) -> (42.31, 0)
  line L104 (41.81, -0.0455) -> (42.31, -0.0455)
  line L105 (41.81, -0.0455) -> (42.31, -0.0455) construction
  line L106 (72.29, 5.5381) -> (72.79, 5.5381) construction
  line L107 (47.39, 5.5381) -> (48.04, 7.0618)
  line L108 (46.24, 7.0618) -> (46.89, 5.5381)
  line L109 (46.24, 7.0618) -> (48.04, 7.0618)
  line L110 (46.24, 7.0618) -> (48.04, 7.0618) construction
  line L111 (46.89, 0.6294) -> (47.39, 0.6294) construction
  line L112 (47.39, -0.0455) -> (47.39, 5.5381)
  line L113 (46.89, 5.5381) -> (46.89, -0.0455)
  line L114 (46.89, 0) -> (47.39, 0)
  line L115 (46.89, -0.0455) -> (47.39, -0.0455)
  line L116 (46.89, -0.0455) -> (47.39, -0.0455) construction
  line L117 (77.37, 5.5381) -> (77.87, 5.5381) construction
  line L118 (52.47, 5.5381) -> (53.12, 7.0618)
  line L119 (51.32, 7.0618) -> (51.97, 5.5381)
  line L120 (51.32, 7.0618) -> (53.12, 7.0618)
  line L121 (51.32, 7.0618) -> (53.12, 7.0618) construction
  line L122 (51.97, 0.6294) -> (52.47, 0.6294) construction
  line L123 (52.47, -0.0455) -> (52.47, 5.5381)
  line L124 (51.97, 5.5381) -> (51.97, -0.0455)
  line L125 (51.97, 0) -> (52.47, 0)
  line L126 (51.97, -0.0455) -> (52.47, -0.0455)
  line L127 (51.97, -0.0455) -> (52.47, -0.0455) construction
  line L128 (82.45, 5.5381) -> (82.95, 5.5381) construction
  line L129 (57.55, 5.5381) -> (58.2, 7.0618)
  line L130 (56.4, 7.0618) -> (57.05, 5.5381)
  line L131 (56.4, 7.0618) -> (58.2, 7.0618)
  line L132 (56.4, 7.0618) -> (58.2, 7.0618) construction
  line L133 (57.05, 0.6294) -> (57.55, 0.6294) construction
  line L134 (57.55, -0.0455) -> (57.55, 5.5381)
  line L135 (57.05, 5.5381) -> (57.05, -0.0455)
  line L136 (57.05, 0) -> (57.55, 0)
  line L137 (57.05, -0.0455) -> (57.55, -0.0455)
  line L138 (57.05, -0.0455) -> (57.55, -0.0455) construction
  line L139 (87.53, 5.5381) -> (88.03, 5.5381) construction
  line L140 (62.63, 5.5381) -> (63.28, 7.0618)
  line L141 (61.48, 7.0618) -> (62.13, 5.5381)
  line L142 (61.48, 7.0618) -> (63.28, 7.0618)
  line L143 (61.48, 7.0618) -> (63.28, 7.0618) construction
  line L144 (62.13, 0.6294) -> (62.63, 0.6294) construction
  line L145 (62.63, -0.0455) -> (62.63, 5.5381)
  line L146 (62.13, 5.5381) -> (62.13, -0.0455)
  line L147 (62.13, 0) -> (62.63, 0)
  line L148 (62.13, -0.0455) -> (62.63, -0.0455)
  line L149 (62.13, -0.0455) -> (62.63, -0.0455) construction
  line L150 (92.61, 5.5381) -> (93.11, 5.5381) construction
  line L151 (31.9, 0) -> (31.9, 7.0618) construction
  point P0 (31.9, -5.7676)
  point P1 (1.42, 7.0618)
  point P2 (1.42, 0.6294)
  point P3 (31.9, 4.1598)
  point P4 (0, 7.0506)
  point P5 (63.8, 7.0506)
  point P6 (6.5, 7.0618)
  point P7 (36.98, 4.1598)
  point P8 (6.5, 0.6294)
  point P9 (6.5, 0)
  point P10 (11.58, 7.0618)
  point P11 (42.06, 4.1598)
  point P12 (11.58, 0.6294)
  point P13 (11.58, 0)
  point P14 (16.66, 7.0618)
  point P15 (47.14, 4.1598)
  point P16 (16.66, 0.6294)
  point P17 (16.66, 0)
  point P18 (21.74, 7.0618)
  point P19 (52.22, 4.1598)
  point P20 (21.74, 0.6294)
  point P21 (21.74, 0)
  point P22 (26.82, 7.0618)
  point P23 (57.3, 4.1598)
  point P24 (26.82, 0.6294)
  point P25 (26.82, 0)
  point P26 (62.38, 4.1598)
  point P27 (31.9, 0.6294)
  point P28 (36.98, 7.0618)
  point P29 (67.46, 4.1598)
  point P30 (36.98, 0.6294)
  point P31 (36.98, 0)
  point P32 (42.06, 7.0618)
  point P33 (72.54, 4.1598)
  point P34 (42.06, 0.6294)
  point P35 (42.06, 0)
  point P36 (47.14, 7.0618)
  point P37 (77.62, 4.1598)
  point P38 (47.14, 0.6294)
  point P39 (47.14, 0)
  point P40 (52.22, 7.0618)
  point P41 (82.7, 4.1598)
  point P42 (52.22, 0.6294)
  point P43 (52.22, 0)
  point P44 (57.3, 7.0618)
  point P45 (87.78, 4.1598)
  point P46 (57.3, 0.6294)
  point P47 (57.3, 0)
  point P48 (62.38, 7.0618)
  point P49 (92.86, 4.1598)
  point P50 (62.38, 0.6294)
  point P51 (62.38, 0)
  point P52 (31.9, 4.1598)
  dimension "d144" = 0.5
  dimension "d145" = 1.8
  dimension "d156" = 5.08
  constraints: 298 end point, 59 point on line, 4 horizontal, 3 midpoint, 2 perpendicular, 2 vertical, 1 parallel, 324 other
  measures "d144" distance between parallel lines of L3 L1
  measures "d145" distance of L4.end L0.start
  measures "d156" distance of L4.end L19.end
extrude "Выдавливание14" cut sketch "Эскиз17" against normal blind 10 contours L5 L4 L3 L17 L1 L0 | L146 L141 L142 L140 L145 L17 | L135 L130 L131 L129 L134 L17 | L124 L119 L120 L118 L123 L17 | L113 L108 L109 L107 L112 L17 | L102 L97 L98 L96 L101 L17 | L91 L86 L87 L85 L90 L17 | L80 L75 L76 L74 L79 L17 | L69 L64 L65 L63 L68 L17 | L58 L53 L54 L52 L57 L17 | L47 L42 L43 L41 L46 L17 | L36 L31 L32 L30 L35 L17 | L25 L20 L21 L19 L24 L17
sketch "Эскиз11" plane through (34.8, -6.95, 0) normal (0, 0, -1) x (-1, 0, 0)
  line L0 (49.8, 0) -> (19.8, 0)
  line L1 (19.8, 0) -> (19.8, 1.5)
  line L2 (19.8, 1.5) -> (49.8, 1.5)
  line L3 (49.8, 1.5) -> (49.8, 0)
  line L4 (67.3, 1.5) -> (2.3, 1.5) projected
  line L5 (0, 0) -> (69.6, 0) projected
  point P0 (34.8, 6.95)
  point P1 (34.8, 0)
  dimension "d67" = 30
  constraints: 8 end point, 2 collinear, 2 parallel, 1 horizontal, 1 midpoint, 1 perpendicular, 1 vertical alignment
  measures "d67" distance between parallel lines of L1 L3
extrude "Выдавливание9" add sketch "Эскиз11" along normal blind 3.5
sketch "Эскиз12" plane through (-32.5, -5.45, 5) normal (0, 1, 0) x (1, 0, 0)
  line L0 (65, 0) -> (0, 0) construction
  line L1 (65, 5) -> (65, 0) construction
  line L2 (0, 5) -> (0, 0) construction
  line L3 (0.18, 0) -> (1.38, 0)
  line L4 (1.38, 0) -> (2, 8.5)
  line L5 (2, 8.5) -> (63, 8.5)
  line L6 (63, 8.5) -> (63.62, 0)
  line L7 (63.62, 0) -> (64.82, 0)
  line L8 (65, 9.5) -> (0, 9.5)
  line L9 (64.82, 0) -> (65, 5)
  line L10 (65, 5) -> (65, 9.5)
  line L11 (0.18, 0) -> (0, 5)
  line L12 (0, 5) -> (0, 9.5)
  line L13 (47.5, 8.5) -> (17.5, 8.5) projected
  point P0 (32.5, 5)
  dimension "d71" = 0.18
  dimension "d72" = 1.2
  dimension "d73" = 2
  dimension "d74" = 1
  constraints: 21 end point, 3 collinear, 3 equal length, 2 vertical, 1 horizontal
  measures "d71" distance from line of L3.start L12
  measures "d72" distance of L3.end L3.start
  measures "d73" horizontal distance of L4.end L2.start
  measures "d74" distance between parallel lines of L8 L13
extrude "Выдавливание10" cut sketch "Эскиз12" against normal through all
sketch "Эскиз13" plane through (0, 0, 0) normal (1, 0, 0) x (0, 1, 0)
  line L0 (-6.95, 0) -> (-6.95, -2)
  line L1 (-6.95, -2) -> (-7.75, 0)
  line L2 (-7.75, 0) -> (-6.95, 0)
  line L3 (-6.95, 0) -> (-6.95, 5) projected
  line L4 (6.95, 0) -> (-6.95, 0) construction
  point P0 (0, 0)
  point P1 (-6.95, -3.5)
  dimension "d77" = 2
  dimension "d78" = 0.8
  constraints: 6 end point, 2 collinear, 1 perpendicular, 1 vertical
  measures "d77" distance from line of L0.end L2
  measures "d78" distance of L1.end L0.start
extrude "Выдавливание11" add sketch "Эскиз13" along normal mid plane 3
sketch "Эскиз14" plane through (2.25, -6.95, 6.5) normal (0, -1, 0) x (1, 0, 0)
  line L0 (-34.75, -11) -> (-34.75, -6.5)
  line L1 (-34.75, -6.5) -> (-35.95, -6.5)
  line L2 (-35.95, -6.5) -> (-35.95, -11)
  line L3 (-35.95, -11) -> (-34.75, -11)
  line L4 (30.25, -11) -> (30.25, -6.5)
  line L5 (30.25, -6.5) -> (31.45, -6.5)
  line L6 (31.45, -6.5) -> (31.45, -11)
  line L7 (31.45, -11) -> (30.25, -11)
  line L8 (-4.5, 0) -> (-36.935, 0) construction
  point P0 (-2.25, -6.5)
  dimension "d83" = 1.2
  dimension "d101" = 11
  constraints: 16 end point, 3 collinear, 3 vertical, 2 coincident, 2 parallel, 2 perpendicular
  measures "d83" distance of L0.end L1.end
  measures "d101" distance between parallel lines of L3 L8
extrude "Выдавливание12" add sketch "Эскиз14" against normal blind 12.4
fillet "Сопряжение6" radius 0.1 9 edges at (34.7425, 6.9, 3.25) (-34.7425, 6.9, 3.25) (34.7425, -6.95, 3.25) (-34.7425, -6.95, 3.25) (-34.685, -0.05, 6.5) (-18.4675, -6.95, 6.5) (18.4675, -6.95, 6.5) (34.685, -0.05, 6.5) (0, 6.85, 6.5)
fillet "Сопряжение7" radius 1.2 2 edges at (-33.1, -6.95, -4.5) (33.1, -6.95, -4.5)
equation "\"d63\" = d62"
equation "\"d62\" = 1.5"
